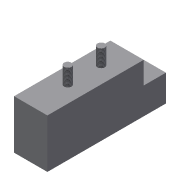
# Autodesk Inventor part: 17-0028-0082
Saved by Autodesk Inventor 2016 SP2 (Build 200236200, 236)
## iProperties
Category: IOP
Company: Universiteit van Amsterdam
Created: 2017-11-24
Part Number: 17-0028-0082
Material: Generic
Document SubType Name: Modeling
Designer: Daan Giesen
Density: 1 g/cm^3
Appearance: Default
Project: Digital PID Loop
Cost Center: 17-0028
User Status: Work in Progress
Authority: Reichsöllner, Lukas
Author: Daan Giesen
Title: Digital PID Loop
Revision Number: A
Autodesk Inventor part; units mm, degrees
ref_plane "YZ Plane" through (0, 0, 0) normal (1, 0, 0) x (0, 1, 0)
ref_plane "XZ Plane" through (0, 0, 0) normal (0, 1, 0) x (-1, 0, 0)
ref_plane "XY Plane" through (0, 0, 0) normal (0, 0, 1) x (1, 0, 0)
sketch "Sketch1" plane through (0, 0, 0) normal (0, 0, 1) x (1, 0, 0)
  line L0 (0, 112) -> (0, -112) construction
  line L1 (-31.5, 0) -> (31.5, 0) construction
  line L2 (-22.5, 80) -> (22.5, 80)
  line L3 (22.5, 80) -> (22.5, -80)
  line L4 (22.5, -80) -> (-22.5, -80)
  line L5 (-22.5, -80) -> (-22.5, 80)
  line L6 (-22.5, 80) -> (22.5, -80) construction
  line L7 (22.5, 80) -> (-22.5, -80) construction
  point P0 (0, 0)
  dimension "d4" = 160
  dimension "d5" = 45
  constraints: 12 end point, 2 midpoint, 2 parallel, 1 horizontal, 1 perpendicular
  measures "d4" distance of L2.end L3.end
  measures "d5" distance of L3.end L4.end
extrude "Extrusion3" add sketch "Sketch1" along normal blind 66
sketch "Sketch2" plane through (0, 0, 66) normal (0, 0, 1) x (1, 0, 0)
  circle A0 centre (0, -30) radius 5
  circle A1 centre (0, 15) radius 5
  line L0 (-22.5, -80) -> (22.5, -80) projected
  point P0 (0, 0)
  dimension "d8" = 10
  dimension "d9" = 50
  dimension "d10" = 45
  constraints: 2 centre point, 1 equal radius
  measures "d8" diameter of A0
  measures "d9" distance from line of L0 A0.centre
  measures "d10" distance of A0.centre A1.centre
extrude "Extrusion4" add sketch "Sketch2" along normal blind 23
thread "Thread1" size "M10x1.5" class "6g" standard "ISO Metric profile" full length
thread "Thread2" size "M10x1.5" class "6g" standard "ISO Metric profile" full length
sketch "Sketch3" plane through (22.5, -80, 0) normal (1, 0, 0) x (0, 0, -1)
  line L0 (0, 160) -> (0, 0) projected
  line L1 (0, 160) -> (-66, 160) projected
  line L2 (-66, 0) -> (-66, 160) projected
  line L3 (0, 0) -> (-66, 0) projected
  line L4 (-66, 160) -> (-36, 160)
  line L5 (-36, 160) -> (-36, 130)
  line L6 (-36, 130) -> (-66, 130)
  line L7 (-66, 130) -> (-66, 160)
  point P0 (0, 80)
  dimension "d17" = 30
  dimension "d18" = 30
  constraints: 8 end point, 2 parallel, 1 horizontal, 1 perpendicular
  measures "d17" distance of L5.end L6.end
  measures "d18" distance of L4.end L5.end
extrude "Extrusion5" cut sketch "Sketch3" against normal through all contours L5 L6 L2 L1
body "Solid3"
